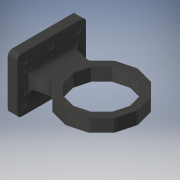
# Autodesk Inventor part: pneumaticholder
Saved by Autodesk Inventor 2019 (Build 230136000, 136)
## iProperties
Created: 2019-01-24
Part Number: pneumaticholder
Material: Generic
Document SubType Name: Modeling
Designer: rachala.rohit
Density: 1 g/cm^3
Appearance: Smooth - Black
Author: rachala.rohit
Autodesk Inventor part; units mm, degrees
ref_plane "YZ Plane" through (0, 0, 0) normal (1, 0, 0) x (0, 1, 0)
ref_plane "XZ Plane" through (0, 0, 0) normal (0, 1, 0) x (-1, 0, 0)
ref_plane "XY Plane" through (0, 0, 0) normal (0, 0, 1) x (1, 0, 0)
sketch "Sketch2" plane through (0, 0, 0) normal (0, 1, 0) x (-1, 0, 0)
  line L0 (0, -19.985) -> (-9.9925, -17.3075)
  line L1 (-9.9925, -17.3075) -> (-17.3075, -9.9925)
  line L2 (-17.3075, -9.9925) -> (-19.985, 0)
  line L3 (-19.985, 0) -> (-17.3075, 9.9925)
  line L4 (-17.3075, 9.9925) -> (-9.9925, 17.3075)
  line L5 (-9.9925, 17.3075) -> (0, 19.985)
  line L6 (0, 19.985) -> (9.9925, 17.3075)
  line L7 (9.9925, 17.3075) -> (17.3075, 9.9925)
  line L8 (17.3075, 9.9925) -> (19.985, 0)
  line L9 (19.985, 0) -> (17.3075, -9.9925)
  line L10 (17.3075, -9.9925) -> (9.9925, -17.3075)
  line L11 (9.9925, -17.3075) -> (0, -19.985)
  line L12 (0, -25.2442) -> (-12.6221, -21.8621)
  line L13 (-12.6221, -21.8621) -> (-21.8621, -12.6221)
  line L14 (-21.8621, -12.6221) -> (-25.2442, 0)
  line L15 (-25.2442, 0) -> (-21.8621, 12.6221)
  line L16 (-21.8621, 12.6221) -> (-12.6221, 21.8621)
  line L17 (-12.6221, 21.8621) -> (0, 25.2442)
  line L18 (0, 25.2442) -> (12.6221, 21.8621)
  line L19 (12.6221, 21.8621) -> (21.8621, 12.6221)
  line L20 (21.8621, 12.6221) -> (25.2442, 0)
  line L21 (25.2442, 0) -> (21.8621, -12.6221)
  line L22 (21.8621, -12.6221) -> (12.6221, -21.8621)
  line L23 (12.6221, -21.8621) -> (0, -25.2442)
  point P0 (0, 0)
  point P1 (0, 0)
  point P2 (0, 0)
  dimension "d1" = 38.608
  dimension "d2" = 5.08
  constraints: 48 end point, 2 coincident, 50 other
  measures "d1" distance between parallel lines of L2 L8
  measures "d2" distance between parallel lines of L11 L23
extrude "Extrusion1" add sketch "Sketch2" along normal blind 8.89
sketch "Sketch3" plane through (0, 8.89, 0) normal (0, 1, 0) x (1, 0, 0)
  line L0 (-25.2442, 0) -> (-21.8621, -12.6221) projected
  line L1 (-21.8621, -12.6221) -> (-35.1484, -16.1822)
  line L2 (-12.6221, 21.8621) -> (-21.8621, 12.6221) projected
  line L3 (-21.8621, 12.6221) -> (-25.2442, 0) projected
  line L4 (-21.8621, 12.6221) -> (-25.2442, 0)
  line L5 (-25.2442, 0) -> (-21.8621, -12.6221)
  line L6 (-21.8621, 12.6221) -> (-35.1484, 16.1822)
  line L7 (-35.1484, 16.1822) -> (-35.1484, -16.1822)
  point P0 (0, 0)
  constraints: 10 end point, 2 perpendicular, 1 collinear, 1 vertical
extrude "Extrusion2" add sketch "Sketch3" against normal blind 8.89
sketch "Sketch5" plane through (-35.1484, 8.89, -16.1822) normal (-1, 0, 0) x (0, 0, 1)
  line L0 (32.3643, -8.89) -> (0, -8.89) projected
  line L1 (32.3643, 0) -> (32.3643, -8.89) projected
  line L2 (40.3145, 14.605) -> (-7.9455, 14.605)
  line L3 (-7.9455, 14.605) -> (-7.9455, -23.495)
  line L4 (-7.9455, -23.495) -> (40.3145, -23.495)
  line L5 (40.3145, -23.495) -> (40.3145, 14.605)
  line L6 (40.3145, 14.605) -> (-7.9455, -23.495) construction
  line L7 (-7.9455, 14.605) -> (40.3145, -23.495) construction
  point P0 (16.1822, -8.89)
  point P1 (16.1845, -4.445)
  dimension "d7" = 4.445
  dimension "d8" = 16.1798
  dimension "d9" = 38.1
  dimension "d10" = 48.26
  constraints: 12 end point, 2 midpoint, 2 parallel, 1 horizontal, 1 perpendicular
  measures "d7" distance from line of L0 point (16.185, -4.445)
  measures "d8" distance from line of point (16.185, -4.445) L1
  measures "d9" distance of L2.end L3.end
  measures "d10" distance of L3.end L4.end
extrude "Extrusion3" add sketch "Sketch5" along normal blind 6.35
fillet "Fillet1" radius 3.175 19 edges at (-35.1484, 4.445, 16.1822) (-35.1484, 8.89, 0) (-35.1484, 4.445, -16.1822) (-35.1484, 0, 0) (-38.3234, -14.605, -24.1276) (-38.3234, 23.495, -24.1276) (-38.3234, 23.495, 24.1324) (-38.3234, -14.605, 24.1324) (12.6221, 4.445, 21.8621) (0, 4.445, 25.2442) (-12.6221, 4.445, 21.8621) (-21.8621, 4.445, 12.6221) (21.8621, 4.445, 12.6221) (25.2442, 4.445, 0) (21.8621, 4.445, -12.6221) (12.6221, 4.445, -21.8621) (0, 4.445, -25.2442) (-12.6221, 4.445, -21.8621) (-21.8621, 4.445, -12.6221)
sketch "Sketch6" plane through (-35.1484, 8.89, -16.1822) normal (1, 0, 0) x (0, 0, -1)
  circle A0 centre (2.4363, -17.399) radius 2.159
  line L0 (-34.8006, -12.065) -> (2.4363, -12.065) projected
  circle A1 centre (-34.8006, -17.399) radius 2.159
  circle A2 centre (-34.8006, 8.509) radius 2.159
  line L1 (2.4363, 3.175) -> (-34.8006, 3.175) projected
  circle A3 centre (2.4363, 8.509) radius 2.159
  circle A4 centre (-16.1822, 8.509) radius 2.159
  circle A5 centre (-16.1822, -17.399) radius 2.159
  point P0 (-16.1822, -8.89)
  dimension "d14" = 4.318
  dimension "d15" = 5.334
  dimension "d16" = 4.318
  dimension "d17" = 5.334
  constraints: 6 centre point
  measures "d14" diameter of A0
  measures "d15" distance from line of L0 A0.centre
  measures "d16" diameter of A2
  measures "d17" distance from line of L1 A2.centre
extrude "Extrusion4" cut sketch "Sketch6" against normal blind 6.35
equation "\"d16\" = d14"
equation "\"d17\" = d15"
body "Solid1"
